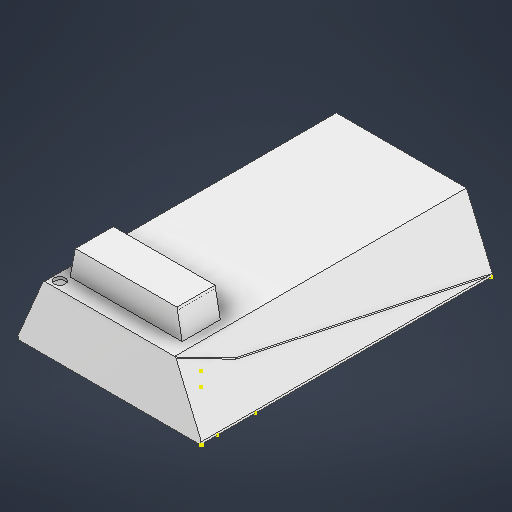
# Autodesk Inventor part: Cover
Saved by Autodesk Inventor 2027 (Build 310192060, 192F)
## iProperties
Created: 2026-06-05
Part Number: Cover
Material: ABS Plastic
Document SubType Name: Modeling
Designer: CatKartikSUPREMEPC
Density: 1.06 g/cm^3
Appearance: Smooth - White
Author: CatKartikSUPREMEPC
Autodesk Inventor part; units mm, degrees
ref_plane "YZ Plane" through (0, 0, 0) normal (1, 0, 0) x (0, 1, 0)
ref_plane "XZ Plane" through (0, 0, 0) normal (0, 1, 0) x (-1, 0, 0)
ref_plane "XY Plane" through (0, 0, 0) normal (0, 0, 1) x (1, 0, 0)
sketch "Sketch1" plane through (0, 0, 0) normal (0, 1, 0) x (-1, 0, 0)
  line L0 (0, 0) -> (200, 0)
  line L1 (200, 0) -> (200, -320)
  line L2 (200, -320) -> (0, -320)
  line L3 (0, -320) -> (0, 0)
  dimension "d0" = 200
  dimension "d1" = 320
  constraints: 8 end point, 2 parallel, 1 horizontal, 1 perpendicular
  measures "d0" distance of L1.end L2.end
  measures "d1" distance of L0.end L1.end
extrude "Extrusion1" add sketch "Sketch1" along normal blind 70
sketch "Sketch2" plane through (-200, 0, 0) normal (0, 0, 1) x (1, 0, 0)
  line L0 (0, 0) -> (0, 70) projected
  line L1 (0, 3) -> (28.4398, 70)
  line L2 (200, 70) -> (0, 70) projected
  line L3 (28.4398, 70) -> (0, 70)
  line L4 (0, 70) -> (0, 3)
  line L5 (0, 0) -> (200, 0) projected
  line L6 (100, 70) -> (100, 0) construction
  line L7 (200, 0) -> (200, 70) projected
  line L8 (200, 3) -> (171.5602, 70)
  line L9 (171.5602, 70) -> (200, 70)
  line L10 (200, 70) -> (200, 3)
  dimension "d4" = 3
  dimension "d5" = 67
  dimension "d6" = 67
  constraints: 14 end point, 4 point on line, 3 collinear, 2 midpoint, 1 perpendicular
  measures "d4" distance of L0.start L1.start
  measures "d5" angle of L5 L1
  measures "d6" angle of L5 L8
extrude "Extrusion2" cut sketch "Sketch2" against normal blind 320 contours L0 L2 L1 | L8 L2 L7
sketch "Sketch3" plane through (0, 0, 0) normal (0, -1, 0) x (1, 0, 0)
  point P0 (0, 0)
shell "Shell1" thickness 15 removed faces 1 at (-66.6667, 0, -106.6667)
sketch "Sketch4" plane through (0, 0, 0) normal (0, -1, 0) x (1, 0, 0)
  circle A0 centre (-7.8764, -158.7609) radius 6
  circle A1 centre (-7.8764, -6.7609) radius 6
  circle A2 centre (-7.8764, -310.7609) radius 6
  circle A3 centre (-192.1236, -158.7609) radius 6
  circle A4 centre (-192.1236, -6.7609) radius 6
  circle A5 centre (-192.1236, -310.7609) radius 6
  point P0 (0, 0)
  dimension "d10" = 12
  dimension "d11" = 12
  dimension "d12" = 152
  dimension "d13" = 12
  dimension "d14" = 152
  constraints: 6 centre point
  measures "d10" diameter of A0
  measures "d11" diameter of A1
  measures "d12" distance of A0.centre A1.centre
  measures "d13" diameter of A2
  measures "d14" distance of A2.centre A0.centre
extrude "Extrusion3" cut sketch "Sketch4" against normal blind 3
sketch "Sketch5" plane through (0, 70, 0) normal (0, 1, 0) x (1, 0, 0)
  point P0 (0, 0)
sketch "Sketch6" plane through (-161.6319, 55, -15) normal (0, -1, 0) x (1, 0, 0)
  point P0 (161.6319, 15)
sketch "Sketch7" plane through (-161.6319, 55, -15) normal (0, -1, 0) x (1, 0, 0)
  line L0 (0, -290) -> (0, 0) projected
  line L1 (123.2638, 0) -> (123.2638, -290) projected
  line L2 (0, -3.1892) -> (123.2638, -3.1892)
  line L3 (123.2638, -3.1892) -> (123.2638, -45.0875)
  line L4 (123.2638, -45.0875) -> (0, -45.0875)
  line L5 (0, -45.0875) -> (0, -3.1892)
  point P0 (161.6319, 15)
  constraints: 8 end point, 2 parallel, 2 point on line, 1 horizontal, 1 perpendicular
extrude "Extrusion4" cut sketch "Sketch7" against normal blind 15
sketch "Sketch13" plane through (0, 70, 0) normal (0, 1, 0) x (1, 0, 0)
  line L0 (-38.3681, 18.1892) -> (-38.3681, 60.0875) projected
  line L1 (-161.6319, 60.0875) -> (-38.3681, 60.0875) projected
  line L2 (-38.3681, 18.1892) -> (-161.6319, 18.1892)
  line L3 (-161.6319, 18.1892) -> (-161.6319, 60.0875)
  line L4 (-161.6319, 60.0875) -> (-38.3681, 60.0875)
  line L5 (-38.3681, 60.0875) -> (-38.3681, 18.1892)
  point P0 (0, 0)
  constraints: 8 end point, 2 parallel, 1 horizontal, 1 perpendicular
extrude "Extrusion7" add sketch "Sketch13" along normal blind 30
sketch "Sketch14" plane through (-161.6319, 70, -18.1892) normal (0, 0, 1) x (1, 0, 0)
  line L0 (0, 30) -> (123.2638, 30) projected
  line L1 (0, 0) -> (0, 30) projected
  line L2 (0, 30) -> (0, 0)
  line L3 (0, 0) -> (5.7383, 30)
  line L4 (5.7383, 30) -> (0, 30)
  line L5 (61.6319, 35.977) -> (61.6319, -1.3966) construction
  line L6 (123.2638, 30) -> (0, 30)
  line L7 (123.2638, 0) -> (123.2638, 30)
  line L8 (123.2638, 0) -> (117.5255, 30)
  point P0 (161.6319, -70)
  constraints: 14 end point, 4 symmetric about line, 2 point on line, 1 collinear, 1 perpendicular, 1 vertical
extrude "Extrusion8" cut sketch "Sketch14" against normal blind 45
sketch "Sketch15" plane through (0, 70, 0) normal (0, -1, 0) x (1, 0, 0)
  line L0 (-38.3681, -60.0875) -> (-38.3681, -18.1892) projected
  line L1 (-38.3681, -60.0875) -> (-161.2693, -60.0875)
  line L2 (-161.2693, -60.0875) -> (-161.2693, -18.1892)
  line L3 (-161.2693, -18.1892) -> (-38.3681, -18.1892)
  line L4 (-38.3681, -18.1892) -> (-38.3681, -60.0875)
  point P0 (0, 0)
  constraints: 8 end point, 2 parallel, 1 horizontal, 1 perpendicular
extrude "Extrusion9" add sketch "Sketch15" along normal blind 15
sketch "Sketch16" plane through (-161.6319, 55, -305) normal (0, -1, 0) x (1, 0, 0)
  line L0 (123.2638, 244.9125) -> (123.2638, 286.8108) projected
  line L1 (123.2638, 244.9125) -> (0.3626, 244.9125)
  line L2 (0.3626, 244.9125) -> (0.3626, 286.8108)
  line L3 (0.3626, 286.8108) -> (123.2638, 286.8108)
  line L4 (123.2638, 286.8108) -> (123.2638, 244.9125)
  point P0 (161.6319, 305)
  constraints: 8 end point, 2 parallel, 1 horizontal, 1 perpendicular
sketch "Sketch17" plane through (0, 100, 0) normal (0, 1, 0) x (1, 0, 0)
  line L0 (-44.1064, 18.1892) -> (-44.1064, 60.0875) projected
  line L1 (-155.8936, 58.8761) -> (-44.1064, 58.8761)
  line L2 (-44.1064, 58.8761) -> (-44.1064, 20.4786)
  line L3 (-44.1064, 20.4786) -> (-155.8936, 20.4786)
  line L4 (-155.8936, 20.4786) -> (-155.8936, 58.8761)
  point P0 (0, 0)
  constraints: 8 end point, 2 parallel, 1 horizontal, 1 perpendicular, 1 point on line
extrude "Extrusion10" cut sketch "Sketch17" against normal blind 100
sketch "Sketch19" plane through (0, 100, 0) normal (0, 1, 0) x (1, 0, 0)
  line L0 (-38.3681, 18.1892) -> (-161.2693, 18.1892) projected
  line L1 (-155.8798, 18.1892) -> (-155.8798, 60.053)
  line L2 (-155.8798, 60.053) -> (-44.1064, 60.053)
  line L3 (-155.8936, 20.4786) -> (-44.1064, 20.4786) projected
  line L4 (-44.1064, 60.053) -> (-44.1064, 20.4786)
  line L5 (-44.1064, 18.1892) -> (-155.8798, 18.1892)
  line L6 (-155.8798, 18.1892) -> (-44.1064, 18.1892)
  line L7 (-44.1064, 18.1892) -> (-44.1064, 60.053)
  point P0 (0, 0)
  point P1 (-155.8798, 20.4786)
  constraints: 12 end point, 3 collinear, 2 perpendicular, 2 point on line, 1 vertical
extrude "Extrusion11" add sketch "Sketch19" against normal blind 3 contours L3 L1 L2 L4
sketch "Sketch23" plane through (-200, 0, 0) normal (0, 0, 1) x (1, 0, 0)
  point P0 (200, 0)
sketch "Sketch25" plane through (-155.8936, 100, -18.1892) normal (0, 0, 1) x (1, 0, 0)
  point P0 (155.8936, -100)
sketch "Sketch28" plane through (-200, 0, 0) normal (0, 0, 1) x (1, 0, 0)
  point P0 (200, 0)
sketch "Sketch30" plane through (0, 0, -320) normal (0, 0, -1) x (-1, 0, 0)
  point P0 (0, 0)
sketch "Sketch31" plane through (0, 0, -320) normal (0, 0, -1) x (-1, 0, 0)
  line L0 (12.5074, 0) -> (35.9715, 61.1475)
  line L1 (35.9715, 61.1475) -> (167.3161, 61.1475)
  line L2 (167.3161, 61.1475) -> (193.8361, -0.2095)
  line L3 (193.8361, -0.2095) -> (199.9941, -0.2095)
  line L4 (198.1236, 3) -> (186.1236, 3) projected
  line L5 (199.9941, -0.2095) -> (199.9941, 3.014)
  line L6 (171.5602, 70) -> (200, 3) projected
  line L7 (199.9941, 3.014) -> (171.5602, 70)
  line L8 (171.5602, 70) -> (28.4398, 70)
  line L9 (28.4398, 70) -> (0, 3) projected
  line L10 (28.4398, 70) -> (0, 3)
  line L11 (0, 3) -> (0, 0)
  line L12 (0, 0) -> (12.5074, 0)
  constraints: 20 end point, 4 perpendicular, 2 collinear, 1 horizontal, 1 parallel
extrude "Extrusion18" add sketch "Sketch31" along normal blind 1
sketch "Sketch32" plane through (-12.5074, 0, -320) normal (0, 0, -1) x (-1, 0, 0)
  line L0 (159.0528, 70) -> (15.9324, 70) projected
  line L1 (87.4926, 70) -> (87.4926, -1.0607) construction
  line L2 (15.9324, 70) -> (-12.5074, 3) projected
  line L3 (-0.6877, 30.8454) -> (180.5483, 30.8454) construction
  line L4 (67.4926, 20.8454) -> (107.4926, 20.8454)
  line L5 (112.4926, 25.8454) -> (112.4926, 35.8454)
  line L6 (107.4926, 40.8454) -> (67.4926, 40.8454)
  line L7 (62.4926, 35.8454) -> (62.4926, 25.8454)
  line L8 (62.4926, 20.8454) -> (112.4926, 40.8454) construction
  line L9 (112.4926, 20.8454) -> (62.4926, 40.8454) construction
  arc A0 (67.4926, 40.8454) -> (62.4926, 35.8454) centre (67.4926, 35.8454) ccw
  arc A1 (112.4926, 35.8454) -> (107.4926, 40.8454) centre (107.4926, 35.8454) ccw
  arc A2 (107.4926, 20.8454) -> (112.4926, 25.8454) centre (107.4926, 25.8454) ccw
  arc A3 (62.4926, 25.8454) -> (67.4926, 20.8454) centre (67.4926, 25.8454) ccw
  point P0 (-12.5074, 0)
  point P1 (87.4926, 30.8454)
  dimension "d63" = 50
  dimension "d64" = 20
  dimension "d65" = 5
  constraints: 16 end point, 11 point on line, 8 point on circle, 8 tangent, 4 centre point, 3 equal radius, 3 midpoint, 2 horizontal, 2 parallel, 1 perpendicular, 1 vertical
  measures "d63" distance of L9.end L8.end
  measures "d64" distance of L8.end L9.start
  measures "d65" radius of A0
extrude "Extrusion19" cut sketch "Sketch32" against normal blind 30
sketch "Sketch33" plane through (-44.1064, 100, -60.0875) normal (0, 0, -1) x (-1, 0, 0)
  point P0 (-44.1064, -100)
sketch "Sketch34" plane through (-44.1064, 100, -60.0875) normal (0, 0, -1) x (-1, 0, 0)
  line L0 (0, 0) -> (111.7873, 0) projected
  line L1 (55.8936, 0) -> (55.8936, -29.6783) construction
  line L2 (-5.7383, -30) -> (0, 0) projected
  line L3 (111.7873, 0) -> (117.5255, -30) projected
  line L4 (85.8936, -25) -> (25.8936, -25)
  line L5 (20.8936, -20) -> (20.8936, -10)
  line L6 (25.8936, -5) -> (85.8936, -5)
  line L7 (90.8936, -10) -> (90.8936, -20)
  line L8 (90.8936, -25) -> (20.8936, -5) construction
  line L9 (20.8936, -25) -> (90.8936, -5) construction
  arc A0 (25.8936, -5) -> (20.8936, -10) centre (25.8936, -10) ccw
  arc A1 (20.8936, -20) -> (25.8936, -25) centre (25.8936, -20) ccw
  arc A2 (85.8936, -25) -> (90.8936, -20) centre (85.8936, -20) ccw
  arc A3 (90.8936, -10) -> (85.8936, -5) centre (85.8936, -10) ccw
  point P0 (-44.1064, -100)
  point P1 (55.8936, -15)
  dimension "d68" = 70
  dimension "d69" = 20
  dimension "d71" = 5
  constraints: 14 end point, 8 point on circle, 8 point on line, 8 tangent, 4 centre point, 3 equal radius, 3 midpoint, 2 parallel, 1 horizontal, 1 perpendicular, 1 vertical
  measures "d68" distance of L8.end L9.end
  measures "d69" distance of L9.start L8.end
  measures "d71" radius of A0
extrude "Extrusion20" cut sketch "Sketch34" against normal blind 15
sketch "Sketch35" plane through (0, 3, 0) normal (0.9205049, 0.3907311, 0) x (0, 0, -1)
  line L0 (320.0001, 0) -> (56.0365, 46.4507)
  line L1 (56.0365, 46.4507) -> (0, 72.3071)
  line L2 (0, 0) -> (0, 72.7861) projected
  line L3 (0, 72.3071) -> (0, 0)
  line L4 (0, 0) -> (320.0001, 0)
  point P0 (0, -2.7615)
  constraints: 8 end point, 1 collinear, 1 perpendicular
extrude "Extrusion21" add sketch "Sketch35" along normal blind 1
fillet "Fillet1" radius 1 1 edges at (-8.1544, 24.7698, -188.0183)
fillet "Fillet2" radius 1 1 edges at (-22.2807, 58.0493, -28.0182)
sketch "Sketch36" plane through (-200, 3, -320) normal (-0.9205049, 0.3907311, 0) x (0, 0, 1)
  line L0 (0, 0) -> (241.9811, 47.0174)
  line L1 (320, 72.7861) -> (320, 0) projected
  line L2 (241.9811, 47.0174) -> (320, 72.7861)
  line L3 (320, 72.7861) -> (320, 0)
  line L4 (-0.0001, 78.1462) -> (320, 78.1462) projected
  line L5 (320, 0) -> (0, 0)
  line L6 (0, -2.7615) -> (320, -2.7615) projected
  point P0 (320, 75.3847)
  constraints: 8 end point, 1 parallel, 1 perpendicular
extrude "Extrusion22" add sketch "Sketch36" along normal blind 1
fillet "Fillet3" radius 1 1 edges at (-177.515, 58.5306, -39.0095)
fillet "Fillet4" radius 1 1 edges at (-191.7349, 25.0306, -199.0095)
sketch "Sketch37" plane through (0, 70, 0) normal (0, 1, 0) x (1, 0, 0)
  circle A0 centre (-163.4398, 8.7457) radius 6
  line L0 (-28.4398, 0) -> (-28.4398, 321) projected
  point P0 (0, 0)
  dimension "d82" = 12
  dimension "d83" = 135
  constraints: 1 centre point
  measures "d82" diameter of A0
  measures "d83" distance from line of L0 A0.centre
extrude "Extrusion23" cut sketch "Sketch37" against normal blind 3
sketch "Sketch38" plane through (-12.5074, 0, -320) normal (0, 0, -1) x (-1, 0, 0)
  line L0 (35.9851, 20.8454) -> (54.1159, 40.8454)
  line L1 (54.1159, 40.8454) -> (35.9851, 40.8454)
  line L2 (35.9851, 40.8454) -> (35.9851, 20.8454)
  line L3 (23.4641, 61.1475) -> (154.8087, 61.1475) projected
  line L4 (89.1364, 61.1475) -> (89.1364, -1.7267) construction
  line L5 (142.2876, 20.8454) -> (124.1569, 40.8454)
  line L6 (124.1569, 40.8454) -> (142.2876, 40.8454)
  line L7 (142.2876, 40.8454) -> (142.2876, 20.8454)
  point P0 (-12.5074, 0)
  constraints: 14 end point, 3 symmetric about line, 1 horizontal, 1 midpoint, 1 perpendicular, 1 vertical
extrude "Extrusion24" cut sketch "Sketch38" against normal blind 20
sketch "Sketch39" plane through (0.9205, 3.3907, 0) normal (0.9205049, 0.3907311, 0) x (0, 0, -1)
  point P0 (0, -2.7615)
sketch "Sketch40" plane through (-28.4398, 70, 0) normal (0.9205049, 0.3907311, 0) x (0, 0, -1)
  point P0 (0, -75.5477)
body "Solid1"
